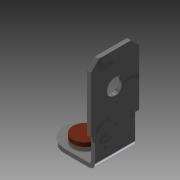
# Autodesk Inventor part: 04
Saved by Autodesk Inventor 2012 (Build 160160000, 160)
## iProperties
Created: 2014-01-28
Part Number: 04
Material: Default
Document SubType Name: Modeling
Designer: Michał
Density: 1 g/cm^3
Author: Michał
Autodesk Inventor part; units mm, degrees
ref_plane "YZ Plane" through (0, 0, 0) normal (1, 0, 0) x (0, 1, 0)
ref_plane "XZ Plane" through (0, 0, 0) normal (0, 1, 0) x (-1, 0, 0)
ref_plane "XY Plane" through (0, 0, 0) normal (0, 0, 1) x (1, 0, 0)
sketch "Sketch1" plane through (0, 0, 0) normal (0, 0, 1) x (1, 0, 0)
  line L0 (-4, -3) -> (4, -3)
  line L1 (4, -3) -> (4, 3)
  line L2 (4, 3) -> (-4, 3)
  line L3 (-4, 3) -> (-4, -3)
  line L4 (-4, 2.5) -> (-10.5, 2.5)
  line L5 (-13, 0) -> (-13, 0)
  line L6 (-10.5, -2.5) -> (-4, -2.5)
  line L7 (-4, -2.5) -> (-4, 2.5)
  arc A0 (-13, 0) -> (-10.5, -2.5) centre (-10.5, 0) ccw
  arc A1 (-10.5, 2.5) -> (-13, 0) centre (-10.5, 0) ccw
  circle A2 centre (-10.5, 0) radius 1
  circle A3 centre (0, 0) radius 1
  point P0 (0, 3)
  point P1 (4, 0)
  point P2 (-13, -2.5)
  point P3 (-13, 2.5)
  point P4 (-4, 0)
  point P5 (-4, 0)
  dimension "d2" = 9
  dimension "d3" = 5
  dimension "d4" = 2.5
  dimension "d5" = 2
  dimension "d6" = 2
  constraints: 16 end point, 5 point on line, 4 centre point, 4 midpoint, 4 parallel, 4 point on circle, 4 tangent, 3 coincident, 2 horizontal, 2 perpendicular, 1 concentric, 1 horizontal alignment, 1 vertical alignment
  measures "d2" distance of L6.end point (-13, -2.5)
  measures "d3" distance of point (-13, -2.5) point (-13, 2.5)
  measures "d4" radius of A0
  measures "d5" diameter of A2
  measures "d6" diameter of A3
extrude "Extrusion1" add sketch "Sketch1" along normal blind 0.5
chamfer "Chamfer1" distance 1 angle 45 2 edges at (4, -3, 0.25) (4, 3, 0.25)
sketch "Sketch2" plane through (0, 0, 0.5) normal (0, 0, 1) x (1, 0, 0)
  arc A0 (-10.5, 2.5) -> (-10.5, -2.5) centre (-10.5, 0) ccw projected
  line L0 (4, 2) -> (4, -2) projected
  line L1 (-7.5, 5.4099) -> (-7.5, -4.87)
  circle A1 centre (-10.5, 0) radius 1 projected
  circle A2 centre (-10.5, 0) radius 1.5
  dimension "d12" = 5.5
  dimension "d15" = 3
  constraints: 2 end point, 1 centre point, 1 coincident, 1 parallel
  measures "d15" diameter of A2
bend part "Bend Part1" radius 0.25 angle 90 line through (-7.5, 5.4099, 0.5) along (0, -1, 0) centre toward (0, 0, 1) moving side (1, 0, 0) both sides no
sketch "Sketch3" plane through (0, 0, 0.5) normal (0, 0, 1) x (1, 0, 0)
  circle A0 centre (-10.5, 0) radius 1 projected
  circle A1 centre (-10.5, 0) radius 1.5
  point P0 (0, 0)
  dimension "d16" = 3
  constraints: 1 centre point, 1 coincident
  measures "d16" diameter of A1
extrude "Extrusion2" add sketch "Sketch3" along normal blind 0.5
sketch "Sketch4" plane through (-10.5, 0, 1) normal (0, 0, 1) x (1, 0, 0)
  circle A0 centre (0, 0) radius 1 projected
  point P0 (10.5, 0)
extrude "Extrusion3" add sketch "Sketch4" against normal up to surface (1 mm away)
body "Solid1"
